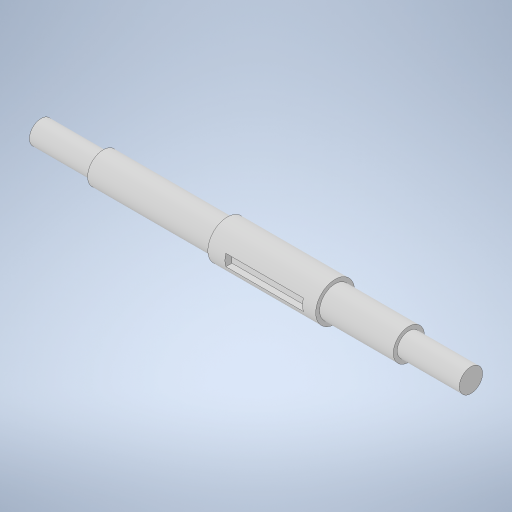
# Autodesk Inventor part: shoulder1_shaft
Saved by Autodesk Inventor 2024 (Build 280153000, 153)
## iProperties
Created: 2025-08-07
Part Number: shoulder1_shaft
Material: 一般
Document SubType Name: Modeling
Designer: HosodaLab2
Density: 1 g/cm^3
Appearance: 既定
Author: HosodaLab2
Autodesk Inventor part; units mm, degrees
ref_plane "YZ Plane" through (0, 0, 0) normal (1, 0, 0) x (0, 1, 0)
ref_plane "XZ Plane" through (0, 0, 0) normal (0, 1, 0) x (-1, 0, 0)
ref_plane "XY Plane" through (0, 0, 0) normal (0, 0, 1) x (1, 0, 0)
sketch "スケッチ1" plane through (0, 0, 0) normal (0, 1, 0) x (-1, 0, 0)
  circle A0 centre (0, 0) radius 5
  dimension "d0" = 10
  constraints: 1 centre point, 1 coincident
  measures "d0" diameter of A0
extrude "押し出し1" add sketch "スケッチ1" along normal blind 27.8
sketch "スケッチ2" plane through (0, 27.8, 0) normal (0, 1, 0) x (1, 0, 0)
  circle A0 centre (0, 0) radius 4
  dimension "d3" = 8
  constraints: 1 centre point, 1 coincident
  measures "d3" diameter of A0
extrude "押し出し2" add sketch "スケッチ2" along normal blind 19
sketch "スケッチ3" plane through (0, 46.8, 0) normal (0, 1, 0) x (1, 0, 0)
  circle A0 centre (0, 0) radius 3
  dimension "d6" = 6
  constraints: 1 centre point, 1 coincident
  measures "d6" diameter of A0
extrude "押し出し3" add sketch "スケッチ3" along normal blind 16
sketch "スケッチ4" plane through (0, 0, 0) normal (0, -1, 0) x (1, 0, 0)
  circle A0 centre (0, 0) radius 4 projected
  circle A1 centre (0, 0) radius 4
  dimension "d9" = 8
  constraints: 1 centre point, 1 coincident
  measures "d9" diameter of A1
extrude "押し出し4" add sketch "スケッチ4" along normal blind 32
sketch "スケッチ5" plane through (0, -32, 0) normal (0, -1, 0) x (1, 0, 0)
  circle A0 centre (0, 0) radius 4 projected
  circle A1 centre (0, 0) radius 3
  dimension "d12" = 6
  constraints: 1 centre point, 1 coincident
  measures "d12" diameter of A1
extrude "押し出し5" add sketch "スケッチ5" along normal blind 16 contours A1
sketch "スケッチ6" plane through (0, 0, 0) normal (0, -1, 0) x (1, 0, 0)
  circle A0 centre (0, 0) radius 5 projected
  point P0 (5, 0)
  constraints: 1 horizontal alignment, 1 other
ref_plane "作業平面1" through (5, 0, 0) normal (1, 0, 0) x (0, 1, 0)
sketch "スケッチ7" plane through (5, 0, 0) normal (1, 0, 0) x (0, 1, 0)
  line L0 (4.4, 1.5) -> (24.4, 1.5)
  line L1 (24.4, 1.5) -> (24.4, -1.5)
  line L2 (24.4, -1.5) -> (4.4, -1.5)
  line L3 (4.4, -1.5) -> (4.4, 1.5)
  line L4 (4.4, 1.5) -> (24.4, -1.5) construction
  line L5 (24.4, 1.5) -> (4.4, -1.5) construction
  line L6 (0, -5) -> (0, 5) projected
  point P0 (0, 0)
  point P1 (14.4, 0)
  dimension "d15" = 20
  dimension "d16" = 3
  dimension "d17" = 4.4
  constraints: 12 end point, 2 midpoint, 2 parallel, 1 horizontal, 1 perpendicular
  measures "d15" distance of L1.end L2.end
  measures "d16" distance of L0.end L1.end
  measures "d17" distance between parallel lines of L6 L3
extrude "押し出し6" cut sketch "スケッチ7" against normal blind 1.8
